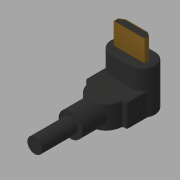
# Autodesk Inventor part: HDMI Mini Right Angle Plug
Saved by Autodesk Inventor 2019 (Build 230136000, 136)
## iProperties
Created: 2019-02-12
Part Number: HDMI Mini Right Angle Plug
Material: Generic
Document SubType Name: Modeling
Designer: Ben
Density: 1 g/cm^3
Appearance: Default
Author: Ben
Autodesk Inventor part; units mm, degrees
ref_plane "YZ Plane" through (0, 0, 0) normal (1, 0, 0) x (0, 1, 0)
ref_plane "XZ Plane" through (0, 0, 0) normal (0, 1, 0) x (-1, 0, 0)
ref_plane "XY Plane" through (0, 0, 0) normal (0, 0, 1) x (1, 0, 0)
sketch "Sketch1" plane through (0, 0, 0) normal (0, 1, 0) x (-1, 0, 0)
  line L0 (7, 3.5) -> (7, -3.5)
  line L1 (-7, -3.5) -> (-7, 3.5)
  line L2 (-7, 3.5) -> (7, -3.5) construction
  line L3 (7, 3.5) -> (-7, -3.5) construction
  line L4 (0, -3.5) -> (0, -5.5) construction
  line L5 (3.375, -9.625) -> (-3.375, -9.625)
  line L6 (-7.5, -5.5) -> (-7.5, -5.5)
  line L7 (-3.375, -1.375) -> (3.375, -1.375) construction
  line L8 (7.5, -5.5) -> (7.5, -5.5)
  line L9 (7.5, -9.625) -> (-7.5, -1.375) construction
  line L10 (-7.5, -9.625) -> (7.5, -1.375) construction
  arc A0 (3.375, -9.625) -> (7.5, -5.5) centre (3.375, -5.5) ccw
  arc A1 (-7.5, -5.5) -> (-3.375, -9.625) centre (-3.375, -5.5) ccw
  line L11 (7, -3.5) -> (6.982717, -3.5)
  line L12 (3.636364, -3.5) -> (-3.636364, -3.5) construction
  line L13 (-6.982717, -3.5) -> (-7, -3.5)
  arc A2 (7.5, -5.5) -> (6.976054, -3.488027) centre (3.375, -5.5) ccw
  arc A3 (5.912734, -2.247996) -> (3.375, -1.375) centre (3.375, -5.5) ccw construction
  arc A4 (-3.375, -1.375) -> (-5.912734, -2.247996) centre (-3.375, -5.5) ccw construction
  arc A5 (-6.976054, -3.488027) -> (-7.5, -5.5) centre (-3.375, -5.5) ccw
  arc A6 (5.5, 3.5) -> (-5.5, 3.5) centre (0, 3.5) ccw
  arc A7 (-5.44475, 2.722375) -> (5.44475, 2.722375) centre (0, 3.5) ccw construction
  line L14 (-7, 3.5) -> (-5.5, 3.5)
  line L15 (5.5, 3.5) -> (7, 3.5)
  point P0 (0, 0)
  dimension "d0" = 14
  dimension "d1" = 7
  dimension "d2" = 2
  dimension "d3" = 15
  dimension "d4" = 8.25
  constraints: 32 end point, 18 point on circle, 16 point on line, 9 parallel, 8 centre point, 6 tangent, 5 midpoint, 3 horizontal, 3 perpendicular, 1 equal radius, 1 vertical
  measures "d0" distance of L0.end L1.start
  measures "d1" distance of L0.start L0.end
  measures "d2" distance of L4.start L4.end
  measures "d3" distance of L9.end L10.end
  measures "d4" distance of L10.start L9.end
extrude "Extrusion1" add sketch "Sketch1" along normal blind 8
sketch "Sketch2" plane through (0, 8, 0) normal (0, 1, 0) x (1, 0, 0)
  line L0 (3.375, 1.375) -> (-3.375, 1.375)
  line L1 (-7.5, 5.5) -> (-7.5, 5.5)
  line L2 (-3.375, 9.625) -> (3.375, 9.625)
  line L3 (7.5, 5.5) -> (7.5, 5.5)
  line L4 (7.5, 1.375) -> (-7.5, 9.625) construction
  line L5 (-7.5, 1.375) -> (7.5, 9.625) construction
  arc A0 (-3.375, 9.625) -> (-7.5, 5.5) centre (-3.375, 5.5) ccw
  arc A1 (-7.5, 5.5) -> (-3.375, 1.375) centre (-3.375, 5.5) ccw
  arc A2 (3.375, 1.375) -> (7.5, 5.5) centre (3.375, 5.5) ccw
  arc A3 (7.5, 5.5) -> (3.375, 9.625) centre (3.375, 5.5) ccw
  point P0 (0, 0)
  point P1 (0, 5.5)
  dimension "d9" = 15
  dimension "d10" = 8.25
  dimension "d11" = 4.125
  constraints: 12 end point, 8 point on circle, 8 point on line, 8 tangent, 4 centre point, 3 equal radius, 2 midpoint, 2 parallel, 1 horizontal, 1 perpendicular
  measures "d9" distance of L4.end L5.end
  measures "d10" distance of L5.start L4.end
  measures "d11" radius of A0
extrude "Extrusion2" add sketch "Sketch2" along normal blind 6.66
fillet "Fillet1" radius 0.5 25 edges at (6.2918, 14.66, -2.5832) (6.2918, 14.66, -8.4168) (0, 14.66, -9.625) (-6.2918, 14.66, -2.5832) (-6.2918, 14.66, -8.4168) (0, 14.66, -1.375) (-7, 8, 0) (-6.25, 8, 3.5) (0, 8, 9) (6.25, 8, 3.5) (7, 8, 0) (0, 0, -9.625) (-7.3686, 0, -4.4671) (-6.2918, 0, -8.4168) (6.2918, 0, -8.4168) (7.3686, 0, -4.4671) (7, 0, 0) (6.25, 0, 3.5) (0, 0, 9) (-6.25, 0, 3.5) (-7, 0, 0) (7, 4, 3.5) (-7, 4, 3.5) (-5.5, 4, 3.5) (5.5, 4, 3.5)
sketch "Sketch3" plane through (-6.5, 0.5, 3.5) normal (0, 0, 1) x (1, 0, 0)
  line L0 (1.01913, 0) -> (1.01913, 7) construction
  line L1 (11.98087, 0) -> (1.01913, 0) construction
  line L2 (11.98087, 7) -> (11.98087, 0) construction
  line L3 (1.01913, 7) -> (11.98087, 7) construction
  line L4 (6.5, 7) -> (6.5, 0) construction
  line L5 (3.125, 0) -> (9.875, 0) construction
  circle A0 centre (6.5, 3.5) radius 4
  point P0 (6.5, -0.5)
  dimension "d15" = 8
  constraints: 3 midpoint, 2 end point, 1 centre point
  measures "d15" diameter of A0
extrude "Extrusion3" add sketch "Sketch3" along normal blind 12
sketch "Sketch4" plane through (0, 4, 15.5) normal (0, 0, 1) x (1, 0, 0)
  circle A0 centre (0, 0) radius 2.5
  point P0 (0, -4)
  dimension "d18" = 5
  constraints: 1 centre point
  measures "d18" diameter of A0
extrude "Extrusion4" add sketch "Sketch4" along normal blind 12
sketch "Sketch5" plane through (0, 14.66, 0) normal (0, 1, 0) x (1, 0, 0)
  arc A0 (3.375, 1.875) -> (3.375, 9.125) centre (3.375, 5.5) ccw construction
  line L0 (-3.375, 9.125) -> (3.375, 9.125) construction
  arc A1 (-3.375, 9.125) -> (-3.375, 1.875) centre (-3.375, 5.5) ccw construction
  line L1 (3.375, 1.875) -> (-3.375, 1.875) construction
  line L2 (-3.375, 9.125) -> (3.375, 9.125) construction
  line L3 (0, 9.125) -> (0, 1.875) construction
  line L4 (3.375, 1.875) -> (-3.375, 1.875) construction
  line L5 (-5.21, 4.25) -> (5.21, 4.25)
  line L6 (5.21, 4.25) -> (5.21, 6.75)
  line L7 (5.21, 6.75) -> (-5.21, 6.75)
  line L8 (-5.21, 6.75) -> (-5.21, 4.25)
  line L9 (-5.21, 4.25) -> (5.21, 6.75) construction
  line L10 (5.21, 4.25) -> (-5.21, 6.75) construction
  line L11 (3.71, 6.75) -> (5.21, 5.75)
  line L12 (3.71, 6.75) -> (5.512776, 6.75) construction
  line L13 (-3.71, 6.75) -> (-5.21, 5.75)
  point P0 (0, 0)
  point P1 (0, 5.5)
  dimension "d21" = 10.42
  dimension "d22" = 2.5
  dimension "d24" = 1.5
  dimension "d25" = 1.5
  dimension "d26" = 1.5
  dimension "d27" = 1.5
  constraints: 20 end point, 5 midpoint, 4 point on line, 2 horizontal, 2 parallel, 1 equal length, 1 perpendicular
  measures "d21" distance of L7.end L6.end
  measures "d22" distance of L6.end L5.end
  measures "d24" distance of L5.end L11.end
  measures "d25" distance of L6.end L11.start
  measures "d26" distance of L5.start L13.end
  measures "d27" distance of L7.end L13.start
extrude "Extrusion5" add sketch "Sketch5" along normal blind 7.15 separate body contours L8 L13 L7 L11 L6 L5
sketch "Sketch6" plane through (0, 21.81, 0) normal (0, 1, 0) x (1, 0, 0)
  line L0 (-5.21, 4.25) -> (5.21, 4.25) construction
  line L1 (5.21, 4.25) -> (5.21, 5.75) construction
  line L2 (5.21, 5.75) -> (3.71, 6.75) construction
  line L3 (3.71, 6.75) -> (-3.71, 6.75) construction
  line L4 (-3.71, 6.75) -> (-5.21, 5.75) construction
  line L5 (-5.21, 5.75) -> (-5.21, 4.25) construction
  line L6 (-3.664584, 6.6) -> (3.664584, 6.6)
  line L7 (3.664584, 6.6) -> (5.06, 5.669722)
  line L8 (5.06, 5.669722) -> (5.06, 4.4)
  line L9 (5.06, 4.4) -> (-5.06, 4.4)
  line L10 (-5.06, 4.4) -> (-5.06, 5.669722)
  line L11 (-5.06, 5.669722) -> (-3.664584, 6.6)
  point P0 (0, 0)
  dimension "d2" = 2
  dimension "d30" = 0.15
  constraints: 12 end point, 5 other
  measures "d30" distance between parallel lines of L3 L6
extrude "Extrusion6" cut sketch "Sketch6" against normal blind 0.15 bodies 2
body "Solid1"
body "Solid2"
